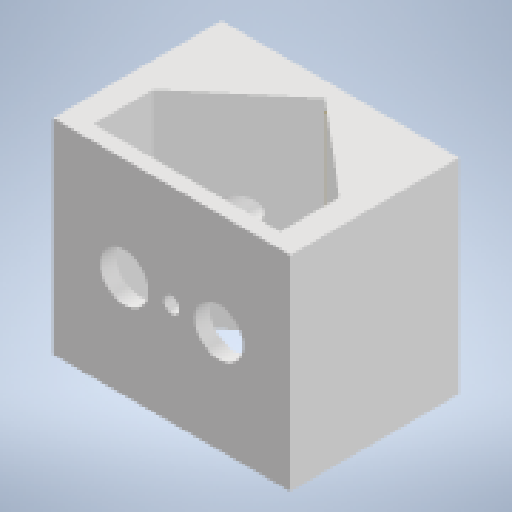
# Autodesk Inventor part: верх крепления маркера
Saved by Autodesk Inventor 2024.2 (Build 282272000, 272)
## iProperties
Created: 2026-01-10
Part Number: верх крепления маркера
Material: Типовые
Document SubType Name: Modeling
Designer: Service
Density: 1 g/cm^3
Appearance: По умолчанию
Author: Service
Autodesk Inventor part; units mm, degrees
ref_plane "YZ Plane" through (0, 0, 0) normal (1, 0, 0) x (0, 1, 0)
ref_plane "XZ Plane" through (0, 0, 0) normal (0, 1, 0) x (-1, 0, 0)
ref_plane "XY Plane" through (0, 0, 0) normal (0, 0, 1) x (1, 0, 0)
ref_plane "РабПлоскость2" through (0, 0, 5) normal (0, 0, 1) x (1, 0, 0)
sketch "Эскиз1" plane through (0, 0, 5) normal (0, 0, 1) x (1, 0, 0)
  circle A0 centre (9.2362, 0) radius 2.15 projected
  circle A1 centre (-9.2362, 0) radius 2.15 projected
  line L0 (-14.2362, -16) -> (14.1136, -16) projected
  arc A2 (14.2362, -15.2592) -> (14.1136, -16) centre (14.9819, -15.7632) ccw projected
  line L1 (14.2362, -15.2592) -> (14.2362, -8.0739) projected
  arc A3 (14.2362, -7.4536) -> (14.2362, -8.0739) centre (15.0811, -7.7638) ccw projected
  line L2 (14.2362, -7.4536) -> (14.2362, 16) projected
  line L3 (14.2362, 16) -> (-14.2362, 16) projected
  line L4 (-14.2362, 16) -> (-14.2362, -16) projected
  circle A4 centre (9.2362, 11) radius 1.6 projected
  circle A5 centre (9.2362, -11) radius 1.6 projected
  circle A6 centre (-9.2362, -11) radius 1.6 projected
  circle A7 centre (-9.2362, 11) radius 1.6 projected
  line L5 (-18.2362, 20) -> (18.2362, 20)
  line L6 (18.2362, 20) -> (18.2362, -20)
  line L7 (18.2362, -20) -> (-18.2362, -20)
  line L8 (-18.2362, -20) -> (-18.2362, 20)
  circle A8 centre (9.2362, 0) radius 1.6
  circle A9 centre (-9.2362, 0) radius 1.6
  dimension "d0" = 4
  dimension "d1" = 4
  dimension "d2" = 4
  dimension "d3" = 4
  constraints: 8 end point, 2 centre point, 2 coincident, 2 equal radius, 2 parallel, 1 horizontal, 1 perpendicular
  measures "d0" distance between parallel lines of L7 L0
  measures "d1" distance between parallel lines of L6 L1
  measures "d2" distance between parallel lines of L8 L4
  measures "d3" distance between parallel lines of L5 L3
extrude "Выдавливание1" add sketch "Эскиз1" along normal blind 3 contours A0 | A1 | L4 L3 L2 A3 L1 A2 L0 | A4 | A5 | A6 | A7 | L5 L6 L7 L8
sketch "Эскиз3" plane through (-18.2362, 20, 5) normal (0, 1, 0) x (1, 0, 0)
  line L0 (0, -3) -> (36.4725, -3) projected
  line L1 (36.4725, -3) -> (36.4725, -18.4215)
  line L2 (36.4725, -18.4215) -> (18.2361, -3)
  line L3 (18.2361, -3) -> (0, -18.4219)
  line L4 (0, -18.4219) -> (0, -3)
  point P0 (18.2362, 5)
  point P1 (18.2361, -3)
  point P2 (18.2361, -3)
  constraints: 8 end point, 1 equal length, 1 parallel, 1 vertical
extrude "Выдавливание2" add sketch "Эскиз3" against normal up to surface (40 mm away)
ref_plane "РабПлоскость4" through (0, 0, 8) normal (0, 0, 1) x (1, 0, 0)
sketch "Эскиз4" plane through (0, 0, 8) normal (0, 0, 1) x (1, 0, 0)
  circle A0 centre (9.2362, 0) radius 1.6 projected
  circle A1 centre (-9.2362, 0) radius 1.6 projected
  circle A2 centre (9.2362, 0) radius 2.7434
  circle A3 centre (-9.2362, 0) radius 2.7434
  point P0 (0, 0)
  constraints: 2 centre point, 2 coincident, 1 equal radius
extrude "Выдавливание3" cut sketch "Эскиз4" along normal blind 14.75 contours A0 | A1 | A2 | A3
sketch "Эскиз5" plane through (0, 0, 5) normal (0, 0, -1) x (-1, 0, 0)
  line L0 (18.2362, 20) -> (18.2362, -20) projected
  line L1 (18.2362, 20) -> (23.2362, 20)
  line L2 (23.2362, 20) -> (23.2362, -20)
  line L3 (23.2362, -20) -> (18.2362, -20)
  line L4 (18.2362, -20) -> (18.2362, 20)
  line L5 (0.0002, -20) -> (-18.2362, -20) projected
  line L6 (-18.2362, -20) -> (-23.2362, -20)
  line L7 (-23.2362, -20) -> (-23.2362, 20)
  line L8 (-23.2362, 20) -> (-18.2362, 20)
  line L9 (-18.2362, 20) -> (-18.2362, -20)
  point P0 (0, 0)
  dimension "d11" = 5
  dimension "d12" = 5
  constraints: 16 end point, 4 parallel, 2 horizontal, 2 perpendicular, 1 point on line
  measures "d11" distance between parallel lines of L2 L0
  measures "d12" distance between parallel lines of L7 L9
extrude "Выдавливание4" add sketch "Эскиз5" against normal blind 30
sketch "Эскиз6" plane through (0, 0, 35) normal (0, 0, 1) x (1, 0, 0)
  line L0 (-23.2362, 20) -> (23.2362, 20)
  line L1 (23.2362, 20) -> (23.2362, -20)
  line L2 (23.2362, -20) -> (-23.2362, -20)
  line L3 (-23.2362, -20) -> (-23.2362, 20)
  circle A0 centre (0, 0) radius 1.55
  line L4 (23.2362, -20) -> (23.2362, 20) projected
  line L5 (23.2362, 20) -> (18.2362, 20) projected
  line L6 (-23.2362, 20) -> (-23.2362, -20) projected
  line L7 (-0.0002, -20) -> (18.2362, -20) projected
  dimension "d15" = 3.1
  constraints: 8 end point, 4 collinear, 2 parallel, 1 centre point, 1 coincident, 1 horizontal, 1 perpendicular
  measures "d15" diameter of A0
extrude "Выдавливание5" add sketch "Эскиз6" along normal blind 3
sketch "Эскиз7" plane through (0, 0, 38) normal (0, 0, 1) x (1, 0, 0)
  circle A0 centre (-9.2362, 0) radius 2.7434 projected
  line L0 (-18.2362, -20) -> (-0.0002, -20) projected
  line L1 (-0.0002, 20) -> (-0.0002, -20) projected
  line L2 (-18.2362, 20) -> (-0.0002, 20) projected
  line L3 (-18.2362, 20) -> (-18.2362, -20) projected
  circle A1 centre (9.2362, 0) radius 2.7434 projected
  line L4 (-0.0002, -20) -> (18.2362, -20) projected
  line L5 (18.2362, 20) -> (18.2362, -20) projected
  line L6 (-0.0002, 20) -> (18.2362, 20) projected
  line L7 (-0.0002, 20) -> (-0.0002, -20) projected
  circle A2 centre (-9.2362, 0) radius 4.6972
  circle A3 centre (9.2362, 0) radius 4.6972
  point P0 (0, 0)
  constraints: 2 centre point, 2 coincident, 1 equal radius
extrude "Выдавливание6" cut sketch "Эскиз7" against normal up to surface (3 mm away) contours A0 | A1 | A2 | A3
